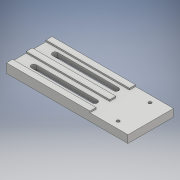
# Autodesk Inventor part: part01
Saved by Autodesk Inventor 2018 (Build 220112000, 112)
## iProperties
Created: 2019-02-06
Part Number: part01
Material: Generic
Document SubType Name: Modeling
Designer: JARVIS
Density: 1 g/cm^3
Appearance: Default
Author: JARVIS
Autodesk Inventor part; units mm, degrees
ref_plane "YZ Plane" through (0, 0, 0) normal (1, 0, 0) x (0, 1, 0)
ref_plane "XZ Plane" through (0, 0, 0) normal (0, 1, 0) x (-1, 0, 0)
ref_plane "XY Plane" through (0, 0, 0) normal (0, 0, 1) x (1, 0, 0)
sketch "Sketch1" plane through (0, 0, 0) normal (0, 0, 1) x (1, 0, 0)
  line L0 (-40, 15) -> (40, 15)
  line L1 (40, 15) -> (40, -15)
  line L2 (40, -15) -> (-40, -15)
  line L3 (-40, -15) -> (-40, 15)
  line L4 (-30, 7) -> (10.125, 7) construction
  line L5 (-30, 5.25) -> (10.125, 5.25)
  line L6 (10.125, 8.75) -> (-30, 8.75)
  arc A0 (-30, 8.75) -> (-30, 5.25) centre (-30, 7) ccw
  arc A1 (10.125, 5.25) -> (10.125, 8.75) centre (10.125, 7) ccw
  line L7 (-30, -7) -> (10.125, -7) construction
  line L8 (-30, -8.75) -> (10.125, -8.75)
  line L9 (10.125, -5.25) -> (-30, -5.25)
  arc A2 (-30, -5.25) -> (-30, -8.75) centre (-30, -7) ccw
  arc A3 (10.125, -8.75) -> (10.125, -5.25) centre (10.125, -7) ccw
  circle A4 centre (29, 10.5) radius 1
  circle A5 centre (29, -10.5) radius 1
  point P0 (0, 0)
  point P1 (-9.9375, 7)
  point P2 (-9.9375, -7)
  point P3 (40, 0)
  point P4 (0, -15)
  dimension "d0" = 21
  dimension "d1" = 11
  dimension "d2" = 30
  dimension "d3" = 2
  dimension "d4" = 4.5
  dimension "d5" = 80
  dimension "d6" = 3.5
  dimension "d7" = 3.5
  dimension "d8" = 10
  dimension "d10" = 10
  dimension "d11" = 8
  dimension "d12" = 8
  dimension "d13" = 18.875
  dimension "d14" = 18.875
  constraints: 24 end point, 8 point on circle, 8 tangent, 6 centre point, 5 parallel, 4 midpoint, 2 horizontal, 2 vertical alignment, 1 equal radius, 1 horizontal alignment, 1 perpendicular
  measures "d0" distance of A4.centre A5.centre
  measures "d1" distance from line of L1 A4.centre
  measures "d2" distance of L0.end L1.end
  measures "d3" diameter of A4
  measures "d4" distance from line of L2 A5.centre
  measures "d5" distance of L1.end L2.end
  measures "d6" distance between parallel lines of L5 L6
  measures "d7" distance between parallel lines of L8 L9
  measures "d8" distance from line of L3 L7.start
  measures "d10" distance from line of L3 L4.start
  measures "d11" distance from line of L2 point (-9.938, -7)
  measures "d12" distance from line of L0 point (-9.938, 7)
  measures "d13" horizontal distance of A4.centre L4.end
  measures "d14" horizontal distance of A5.centre L7.end
extrude "Extrusion1" add sketch "Sketch1" along normal blind 5
sketch "Sketch2" plane through (0, 0, 5) normal (0, 0, 1) x (1, 0, 0)
  line L0 (-40, 15) -> (15, 15)
  line L1 (15, 15) -> (15, 11)
  line L2 (15, 11) -> (-40, 11)
  line L3 (-40, 11) -> (-40, 15)
  line L4 (-40, 2) -> (15, 2)
  line L5 (15, 2) -> (15, -2)
  line L6 (15, -2) -> (-40, -2)
  line L7 (-40, -2) -> (-40, 2)
  line L8 (-40, 15) -> (-40, -15) projected
  line L9 (-40, -15) -> (40, -15) projected
  line L10 (-40, -11) -> (15, -11)
  line L11 (15, -11) -> (15, -15)
  line L12 (15, -15) -> (-40, -15)
  line L13 (-40, -15) -> (-40, -11)
  point P0 (0, 0)
  point P1 (15, 0)
  dimension "d17" = 4
  dimension "d18" = 4
  dimension "d19" = 4
  dimension "d20" = 55
  constraints: 24 end point, 6 parallel, 5 point on line, 3 horizontal, 3 perpendicular, 1 horizontal alignment, 1 midpoint
  measures "d17" distance between parallel lines of L0 L2
  measures "d18" distance between parallel lines of L4 L6
  measures "d19" distance between parallel lines of L10 L9
  measures "d20" distance between parallel lines of L1 L3
extrude "Extrusion2" add sketch "Sketch2" along normal blind 1
chamfer "Chamfer1" distance 2 angle 45 8 edges at (-9.9375, 5.25, 0) (11.875, 7, 0) (-9.9375, 8.75, 0) (-31.75, 7, 0) (-9.9375, -8.75, 0) (11.875, -7, 0) (-9.9375, -5.25, 0) (-31.75, -7, 0)
equation "\"d10\" = d8"
equation "\"d12\" = d11"
equation "\"d14\" = d13"
equation "\"d18\" = d17"
equation "\"d19\" = d17"
body "Solid1"
